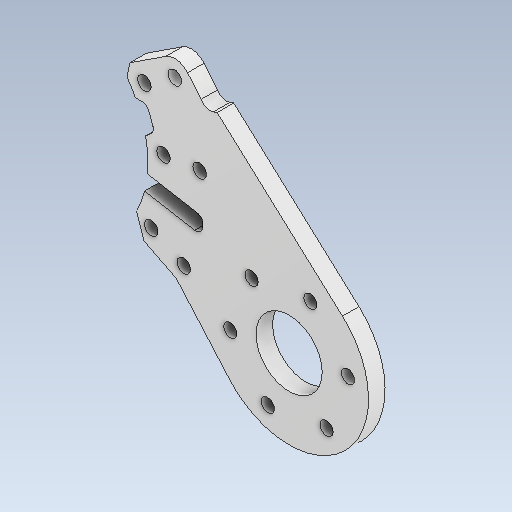
# Autodesk Inventor part: motor_h_5_m
Saved by Autodesk Inventor 2020 (Build 240168000, 168)
## iProperties
Created: 2020-08-09
Part Number: motor_h_5_m
Material: ABS Plastic
Document SubType Name: Modeling
Designer: psrobotics
Density: 1.06 g/cm^3
Appearance: Smooth - White
Author: psrobotics
Autodesk Inventor part; units mm, degrees
ref_plane "YZ Plane" through (0, 0, 0) normal (1, 0, 0) x (0, 1, 0)
ref_plane "XZ Plane" through (0, 0, 0) normal (0, 1, 0) x (-1, 0, 0)
ref_plane "XY Plane" through (0, 0, 0) normal (0, 0, 1) x (1, 0, 0)
sketch "Sketch1" plane through (0, 0, 0) normal (0, 0, 1) x (1, 0, 0)
  circle A0 centre (38.293295, 9.815487) radius 2
  circle A1 centre (49.630187, -4.165746) radius 2
  circle A2 centre (43.190531, -20.974399) radius 2
  circle A3 centre (25.413982, -23.801819) radius 2
  circle A4 centre (14.077089, -9.820586) radius 2
  circle A5 centre (20.516746, 6.988067) radius 2
  circle A6 centre (-68.06383, 51.925322) radius 2.05
  circle A7 centre (-53.750024, 56.410289) radius 2.05
  circle A8 centre (-39.436217, 60.895257) radius 2.05
  line L0 (-78.674955, 0.620135) -> (-78.625805, -1.541882)
  arc A9 (-81.821918, -3.189859) -> (-78.625805, -1.541882) centre (-80.625288, -1.587337) ccw
  line L1 (-81.821918, -3.189859) -> (-83.791584, -1.719076)
  arc A10 (-83.272261, 1.765269) -> (-83.791584, -1.719076) centre (-82.594954, -0.116554) ccw
  line L2 (-83.272261, 1.765269) -> (-81.351745, 2.456502)
  arc A11 (-78.674955, 0.620135) -> (-81.351745, 2.456502) centre (-80.674438, 0.574679) ccw
  line L3 (-1.403552, -3.334837) -> (-3.616041, -5.971578)
  arc A12 (-7.147613, -4.640548) -> (-3.616041, -5.971578) centre (-5.148129, -4.686003) ccw
  line L4 (-7.147613, -4.640548) -> (-7.068079, -1.142036)
  arc A13 (-4.319383, 0.666876) -> (-7.068079, -1.142036) centre (-5.068596, -1.187492) ccw
  line L5 (-4.319383, 0.666876) -> (-2.186427, -0.194894)
  arc A14 (-1.403552, -3.334837) -> (-2.186427, -0.194894) centre (-2.935641, -2.049262) ccw
  arc A15 (-3.40999, 48.096726) -> (-8.055894, 53.961981) centre (-42.851487, 21.62753) ccw
  arc A16 (-4.401032, 43.826911) -> (-3.40999, 48.096726) centre (-5.901032, 46.424987) ccw
  line L6 (-4.401032, 43.826911) -> (-10.914048, 40.066619)
  arc A17 (-14.881949, 40.958979) -> (-10.914048, 40.066619) centre (-12.414048, 42.664695) ccw
  arc A18 (-14.881949, 40.958979) -> (-17.367883, 44.134994) centre (-42.851487, 21.62753) ccw
  arc A19 (-17.417463, 48.04931) -> (-17.367883, 44.134994) centre (-15.11933, 46.120947) ccw
  line L7 (-17.417463, 48.04931) -> (-12.551644, 53.848168)
  arc A20 (-8.055894, 53.961981) -> (-12.551644, 53.848168) centre (-10.25351, 51.919805) ccw
  arc A21 (2.289134, 6.843271) -> (4.050714, 14.115304) centre (-42.851487, 21.62753) ccw
  arc A22 (-1.685672, 4.995462) -> (2.289134, 6.843271) centre (-0.561853, 7.777013) ccw
  line L8 (-1.685672, 4.995462) -> (-8.658636, 7.812722)
  arc A23 (-10.39833, 11.488862) -> (-8.658636, 7.812722) centre (-7.534816, 10.594273) ccw
  arc A24 (-10.39833, 11.488862) -> (-9.42609, 15.403155) centre (-42.851487, 21.62753) ccw
  arc A25 (-6.372092, 17.852118) -> (-9.42609, 15.403155) centre (-6.47679, 14.853945) ccw
  line L9 (-6.372092, 17.852118) -> (1.193168, 17.587933)
  arc A26 (4.050714, 14.115304) -> (1.193168, 17.587933) centre (1.08847, 14.589761) ccw
  line L10 (-77.55058, 9.138616) -> (-84.626781, 6.591747)
  arc A27 (-88.527544, 8.591129) -> (-84.626781, 6.591747) centre (-85.642741, 9.41448) ccw
  arc A28 (-90.338505, 22.73799) -> (-88.527544, 8.591129) centre (-42.851487, 21.62753) ccw
  arc A29 (-87.067158, 25.655485) -> (-90.338505, 22.73799) centre (-87.339325, 22.667856) ccw
  line L11 (-87.067158, 25.655485) -> (-79.577588, 24.973201)
  arc A30 (-76.849895, 21.956541) -> (-79.577588, 24.973201) centre (-79.849755, 21.985572) ccw
  arc A31 (-76.849895, 21.956541) -> (-75.670724, 12.745094) centre (-42.851487, 21.62753) ccw
  arc A32 (-77.55058, 9.138616) -> (-75.670724, 12.745094) centre (-78.566539, 11.96135) ccw
  line L12 (1.367666, 22.584887) -> (-6.197594, 22.849072)
  arc A33 (-9.073322, 25.505106) -> (-6.197594, 22.849072) centre (-6.092896, 25.847245) ccw
  arc A34 (-9.073322, 25.505106) -> (-9.770146, 29.477684) centre (-42.851487, 21.62753) ccw
  arc A35 (-7.778256, 33.023514) -> (-9.770146, 29.477684) centre (-6.851205, 30.170344) ccw
  line L13 (-7.778256, 33.023514) -> (-0.625756, 35.347502)
  arc A36 (3.210472, 33.226926) -> (-0.625756, 35.347502) centre (0.301295, 32.494333) ccw
  arc A37 (4.460489, 25.849725) -> (3.210472, 33.226926) centre (-42.851487, 21.62753) ccw
  arc A38 (1.367666, 22.584887) -> (4.460489, 25.849725) centre (1.472364, 25.58306) ccw
  line L14 (-78.07943, 32.535875) -> (-85.263481, 34.760419)
  arc A39 (-87.175511, 38.704735) -> (-85.263481, 34.760419) centre (-84.376099, 37.626174) ccw
  arc A40 (-83.421221, 46.332726) -> (-87.175511, 38.704735) centre (-42.851487, 21.62753) ccw
  arc A41 (-79.129404, 47.223677) -> (-83.421221, 46.332726) centre (-80.858922, 44.772398) ccw
  line L15 (-79.129404, 47.223677) -> (-72.984388, 42.888016)
  arc A42 (-72.130466, 38.911666) -> (-72.984388, 42.888016) centre (-74.713906, 40.436737) ccw
  arc A43 (-72.130466, 38.911666) -> (-74.407679, 34.284812) centre (-42.851487, 21.62753) ccw
  arc A44 (-78.07943, 32.535875) -> (-74.407679, 34.284812) centre (-77.192048, 35.401631) ccw
  line L16 (-16.381866, 57.062106) -> (-21.247685, 51.263248)
  arc A45 (-25.111143, 50.632361) -> (-21.247685, 51.263248) centre (-23.545819, 53.191611) ccw
  arc A46 (-25.111143, 50.632361) -> (-28.670585, 52.52902) centre (-42.851487, 21.62753) ccw
  arc A47 (-30.238407, 56.281682) -> (-28.670585, 52.52902) centre (-27.419329, 55.255622) ccw
  line L17 (-30.238407, 56.281682) -> (-27.666216, 63.348719)
  arc A48 (-23.633362, 65.06615) -> (-27.666216, 63.348719) centre (-24.847138, 62.322658) ccw
  arc A49 (-17.050461, 61.509319) -> (-23.633362, 65.06615) centre (-42.851487, 21.62753) ccw
  arc A50 (-16.381866, 57.062106) -> (-17.050461, 61.509319) centre (-18.679999, 58.990469) ccw
  line L18 (-27.378641, 16.14178) -> (-17.659555, 17.673703)
  arc A51 (-15.959154, 15.878407) -> (-17.659555, 17.673703) centre (-17.426008, 16.191996) ccw
  arc A52 (-19.770492, 6.677023) -> (-15.959154, 15.878407) centre (-42.851487, 21.62753) ccw
  arc A53 (-22.242323, 6.609923) -> (-19.770492, 6.677023) centre (-21.029455, 7.492505) ccw
  line L19 (-22.242323, 6.609923) -> (-28.031522, 14.565587)
  arc A54 (-27.378641, 16.14178) -> (-28.031522, 14.565587) centre (-27.222943, 15.153976) ccw
  line L20 (-35.789544, 6.807565) -> (-27.833879, 1.018366)
  arc A55 (-27.90098, -1.453465) -> (-27.833879, 1.018366) centre (-28.716462, -0.194501) ccw
  arc A56 (-37.102364, -5.264803) -> (-27.90098, -1.453465) centre (-42.851487, 21.62753) ccw
  arc A57 (-38.897659, -3.564402) -> (-37.102364, -5.264803) centre (-37.415952, -3.797948) ccw
  line L21 (-38.897659, -3.564402) -> (-37.365737, 6.154685)
  arc A58 (-35.789544, 6.807565) -> (-37.365737, 6.154685) centre (-36.377932, 5.998987) ccw
  line L22 (-48.337237, 6.154685) -> (-46.805314, -3.564402)
  arc A59 (-48.60061, -5.264803) -> (-46.805314, -3.564402) centre (-48.287022, -3.797948) ccw
  arc A60 (-57.801994, -1.453465) -> (-48.60061, -5.264803) centre (-42.851487, 21.62753) ccw
  arc A61 (-57.869095, 1.018366) -> (-57.801994, -1.453465) centre (-56.986512, -0.194501) ccw
  line L23 (-57.869095, 1.018366) -> (-49.91343, 6.807565)
  arc A62 (-48.337237, 6.154685) -> (-49.91343, 6.807565) centre (-49.325042, 5.998987) ccw
  line L24 (-57.671452, 14.565587) -> (-63.460651, 6.609923)
  arc A63 (-65.932482, 6.677023) -> (-63.460651, 6.609923) centre (-64.673519, 7.492505) ccw
  arc A64 (-69.74382, 15.878407) -> (-65.932482, 6.677023) centre (-42.851487, 21.62753) ccw
  arc A65 (-68.043419, 17.673703) -> (-69.74382, 15.878407) centre (-68.276966, 16.191996) ccw
  line L25 (-68.043419, 17.673703) -> (-58.324333, 16.14178)
  arc A66 (-57.671452, 14.565587) -> (-58.324333, 16.14178) centre (-58.48003, 15.153976) ccw
  line L26 (-58.324333, 27.11328) -> (-68.043419, 25.581358)
  arc A67 (-69.74382, 27.376654) -> (-68.043419, 25.581358) centre (-68.276966, 27.063065) ccw
  arc A68 (-65.932482, 36.578038) -> (-69.74382, 27.376654) centre (-42.851487, 21.62753) ccw
  arc A69 (-63.460651, 36.645138) -> (-65.932482, 36.578038) centre (-64.673519, 35.762555) ccw
  line L27 (-63.460651, 36.645138) -> (-57.671452, 28.689474)
  arc A70 (-58.324333, 27.11328) -> (-57.671452, 28.689474) centre (-58.48003, 28.101085) ccw
  line L28 (-49.91343, 36.447495) -> (-57.869095, 42.236695)
  arc A71 (-57.801994, 44.708525) -> (-57.869095, 42.236695) centre (-56.986512, 43.449562) ccw
  arc A72 (-48.60061, 48.519864) -> (-57.801994, 44.708525) centre (-42.851487, 21.62753) ccw
  arc A73 (-46.805314, 46.819462) -> (-48.60061, 48.519864) centre (-48.287022, 47.053009) ccw
  line L29 (-46.805314, 46.819462) -> (-48.337237, 37.100376)
  arc A74 (-49.91343, 36.447495) -> (-48.337237, 37.100376) centre (-49.325042, 37.256074) ccw
  line L30 (-37.365737, 37.100376) -> (-38.897659, 46.819462)
  arc A75 (-37.102364, 48.519864) -> (-38.897659, 46.819462) centre (-37.415952, 47.053009) ccw
  arc A76 (-27.90098, 44.708525) -> (-37.102364, 48.519864) centre (-42.851487, 21.62753) ccw
  arc A77 (-27.833879, 42.236695) -> (-27.90098, 44.708525) centre (-28.716462, 43.449562) ccw
  line L31 (-27.833879, 42.236695) -> (-35.789544, 36.447495)
  arc A78 (-37.365737, 37.100376) -> (-35.789544, 36.447495) centre (-36.377932, 37.256074) ccw
  line L32 (-28.031522, 28.689474) -> (-22.242323, 36.645138)
  arc A79 (-19.770492, 36.578038) -> (-22.242323, 36.645138) centre (-21.029455, 35.762555) ccw
  arc A80 (-15.959154, 27.376654) -> (-19.770492, 36.578038) centre (-42.851487, 21.62753) ccw
  arc A81 (-17.659555, 25.581358) -> (-15.959154, 27.376654) centre (-17.426008, 27.063065) ccw
  line L33 (-17.659555, 25.581358) -> (-27.378641, 27.11328)
  arc A82 (-28.031522, 28.689474) -> (-27.378641, 27.11328) centre (-27.222943, 28.101085) ccw
  circle A83 centre (-58.851487, 21.62753) radius 2
  circle A84 centre (-26.851487, 21.62753) radius 2
  circle A85 centre (-32.244885, 11.020929) radius 1.5
  circle A86 centre (-53.458089, 32.234132) radius 1.5
  circle A87 centre (-53.458089, 11.020929) radius 1.5
  circle A88 centre (-32.244885, 32.234132) radius 1.5
  circle A89 centre (-42.851487, 5.62753) radius 2
  circle A90 centre (-42.851487, 37.62753) radius 2
  circle A91 centre (-42.851487, 21.62753) radius 12
  circle A92 centre (7.70065, 40.027004) radius 1.55
  circle A93 centre (-84.475204, 56.808721) radius 1.55
  circle A94 centre (-97.005285, 15.494334) radius 1.55
  circle A95 centre (-90.147142, -5.453293) radius 1.55
  circle A96 centre (-95.005612, 37.445154) radius 1.55
  circle A97 centre (-33.50983, 74.606702) radius 1.55
  circle A98 centre (-1.641007, -12.952168) radius 1.55
  line L34 (-73.415646, -10.729473) -> (-73.624099, -1.560071)
  arc A99 (-66.796705, 1.359267) -> (-73.624099, -1.560071) centre (-69.625132, -1.46916) ccw
  line L35 (-66.796705, 1.359267) -> (-54.272781, -11.164658)
  line L36 (-31.937943, -11.672407) -> (-54.272781, -11.164658)
  line L37 (-31.937943, -11.672407) -> (-18.906268, 1.359267)
  arc A100 (-12.078875, -1.560071) -> (-18.906268, 1.359267) centre (-16.077841, -1.46916) ccw
  line L38 (-12.078875, -1.560071) -> (-12.318903, -12.118417)
  line L39 (-8.896198, -12.196228) -> (-12.318903, -12.118417)
  arc A101 (-7.546122, -12.763059) -> (-8.896198, -12.196228) centre (-8.941653, -14.195711) ccw
  line L40 (-4.169882, -16.05182) -> (-7.546122, -12.763059)
  line L41 (-1.14798, -18.587496) -> (-4.169882, -16.05182)
  line L42 (-1.14798, -18.587496) -> (22.104815, -28.923976)
  arc A102 (22.104815, -28.923976) -> (47.979301, 10.782182) centre (31.853638, -6.993166) ccw
  line L43 (47.979301, 10.782182) -> (10.09134, 45.153855)
  line L44 (8.937474, 44.733882) -> (10.09134, 45.153855)
  arc A103 (5.239682, 46.188463) -> (8.937474, 44.733882) centre (7.911414, 47.55296) ccw
  arc A104 (5.239682, 46.188463) -> (-1.114838, 55.891974) centre (-42.851487, 21.62753) ccw
  arc A105 (-1.795079, 57.715969) -> (-1.114838, 55.891974) centre (1.203865, 57.795554) ccw
  line L45 (-14.440683, 68.326891) -> (-1.795079, 57.715969)
  arc A106 (-16.35509, 68.680064) -> (-14.440683, 68.326891) centre (-14.883068, 71.294094) ccw
  arc A107 (-16.35509, 68.680064) -> (-27.014634, 73.253048) centre (-42.851487, 21.62753) ccw
  arc A108 (-29.089232, 76.642077) -> (-27.014634, 73.253048) centre (-26.134808, 76.121132) ccw
  line L46 (-28.876006, 77.85134) -> (-29.089232, 76.642077)
  line L47 (-36.754468, 79.240526) -> (-28.876006, 77.85134)
  line L48 (-37.439477, 75.355644) -> (-36.754468, 79.240526)
  line L49 (-37.858542, 71.195346) -> (-37.439477, 75.355644)
  arc A109 (-39.248649, 69.487857) -> (-37.858542, 71.195346) centre (-39.848472, 71.395791) ccw
  line L50 (-76.775677, 57.689962) -> (-39.248649, 69.487857)
  arc A110 (-78.666553, 58.07042) -> (-76.775677, 57.689962) centre (-77.3755, 59.597896) ccw
  line L51 (-84.105762, 62.667748) -> (-78.666553, 58.07042)
  line L52 (-89.730392, 56.013112) -> (-84.105762, 62.667748)
  line L53 (-87.956721, 54.513969) -> (-89.730392, 56.013112)
  arc A111 (-87.590763, 51.866531) -> (-87.956721, 54.513969) centre (-89.247774, 52.986494) ccw
  arc A112 (-87.590763, 51.866531) -> (-92.550473, 42.746498) centre (-42.851487, 21.62753) ccw
  arc A113 (-94.971639, 41.614769) -> (-92.550473, 42.746498) centre (-94.391176, 43.528682) ccw
  line L54 (-97.194033, 42.288791) -> (-94.971639, 41.614769)
  line L55 (-99.515886, 34.633139) -> (-97.194033, 42.288791)
  line L56 (-97.293492, 33.959118) -> (-99.515886, 34.633139)
  arc A114 (-95.908867, 31.673145) -> (-97.293492, 33.959118) centre (-97.873956, 32.045205) ccw
  arc A115 (-95.908867, 31.673145) -> (-96.850692, 21.334544) centre (-42.851487, 21.62753) ccw
  arc A116 (-98.625591, 19.336397) -> (-96.850692, 21.334544) centre (-98.850663, 21.323693) ccw
  line L57 (-100.933195, 19.075049) -> (-98.625591, 19.336397)
  line L58 (-100.032909, 11.125868) -> (-100.933195, 19.075049)
  line L59 (-97.725305, 11.387216) -> (-100.032909, 11.125868)
  arc A117 (-95.548493, 9.836621) -> (-97.725305, 11.387216) centre (-97.500234, 9.399921) ccw
  arc A118 (-95.548493, 9.836621) -> (-92.318381, -0.029487) centre (-42.851487, 21.62753) ccw
  arc A119 (-93.156696, -2.567219) -> (-92.318381, -0.029487) centre (-94.150488, -0.831599) ccw
  line L60 (-95.172061, -3.721188) -> (-93.156696, -2.567219)
  line L61 (-88.995524, -14.508281) -> (-95.172061, -3.721188)
  line L62 (-82.535958, -10.809624) -> (-88.995524, -14.508281)
  arc A120 (-81.496711, -10.545761) -> (-82.535958, -10.809624) centre (-81.542166, -12.545245) ccw
  line L63 (-73.415646, -10.729473) -> (-81.496711, -10.545761)
  circle A121 centre (0, 0) radius 2.05
  circle A122 centre (-9.820132, 4.956309) radius 2.05
  circle A123 centre (4.81279, 27.294689) radius 2.05
  circle A124 centre (-6.110273, 25.995965) radius 2.05
  circle A125 centre (-2.695753, 47.924241) radius 2.05
  circle A126 centre (-11.898108, 41.897912) radius 2.05
  circle A127 centre (31.853638, -6.993166) radius 24
  line L64 (0, 0) -> (-9.820132, 4.956309) construction
  line L65 (2.252868, 4.463697) -> (-7.567265, 9.420006)
  line L66 (-12.073, 0.492612) -> (-2.252868, -4.463697)
  arc A128 (-2.252868, -4.463697) -> (2.252868, 4.463697) centre (0, 0) ccw
  arc A129 (-7.567265, 9.420006) -> (-12.073, 0.492612) centre (-9.820132, 4.956309) ccw
  line L67 (-13.628948, 58.787181) -> (-11.330815, 56.858819)
  line L68 (-13.628948, 58.787181) -> (-23.832196, 46.627425)
  spline S0 degree 3 poles (-21.534062, 44.699062) (-21.903382, 45.038051) (-22.279634, 45.368174) (-22.661708, 45.688772) (-23.043782, 46.00937) (-23.434225, 46.322581) (-23.832196, 46.627425) knots 0 0 0 0 0.5 0.5 0.5 1 1 1 1
  line L69 (-21.534062, 44.699062) -> (-11.330815, 56.858819)
  line L70 (3.940984, 14.899895) -> (3.42004, 11.945472)
  line L71 (-11.691298, 17.656288) -> (3.940984, 14.899895)
  spline S1 degree 3 poles (-12.212242, 14.701865) (-12.103331, 15.191187) (-12.00556, 15.682104) (-11.918951, 16.17329) (-11.832342, 16.664475) (-11.756315, 17.159214) (-11.691298, 17.656288) knots 0 0 0 0 0.5 0.5 0.5 1 1 1 1
  line L72 (3.42004, 11.945472) -> (-12.212242, 14.701865)
  line L73 (-2.252868, -4.463697) -> (13.793156, -22.798829)
  line L74 (4.81279, 27.294689) -> (-6.110273, 25.995965) construction
  line L75 (4.222461, 32.259718) -> (-6.700602, 30.960994)
  line L76 (-5.519944, 21.030937) -> (5.403119, 22.329661)
  arc A130 (5.403119, 22.329661) -> (4.222461, 32.259718) centre (4.81279, 27.294689) ccw
  arc A131 (-6.700602, 30.960994) -> (-5.519944, 21.030937) centre (-6.110273, 25.995965) ccw
  line L77 (-2.695753, 47.924241) -> (-11.898108, 41.897912) construction
  line L78 (-5.434993, 52.10713) -> (-14.637349, 46.080801)
  line L79 (-9.158868, 37.715023) -> (0.043488, 43.741352)
  arc A132 (0.043488, 43.741352) -> (-5.434993, 52.10713) centre (-2.695753, 47.924241) ccw
  arc A133 (-14.637349, 46.080801) -> (-9.158868, 37.715023) centre (-11.898108, 41.897912) ccw
  circle A134 centre (-42.851487, 21.62753) radius 32
  line L80 (5.239682, 46.188463) -> (1.15286, 51.116134)
  circle A135 centre (-42.851487, 21.62753) radius 48
  line L81 (4.81279, 27.294689) -> (7.000507, 31.790676)
  line L82 (7.000507, 31.790676) -> (42.354681, 14.587568)
  circle A136 centre (-42.851487, 21.62753) radius 50.87741
  point P0 (0, 0)
  point P1 (-4.910066, 2.478155)
  point P2 (-0.648742, 26.645327)
  point P3 (-7.296931, 44.911077)
  point P4 (-16.080997, 39.158671)
  point P5 (-14.283829, 7.209177)
  dimension "d0" = 48
  dimension "d1" = 10
  dimension "d2" = 10
  dimension "d3" = 10
  dimension "d4" = 64
  constraints: 32 end point, 16 point on circle, 15 tangent, 8 centre point, 4 coincident, 3 midpoint, 3 parallel, 1 perpendicular, 6 other
  measures "d0" diameter of A127
  measures "d1" diameter of A129
  measures "d2" diameter of A131
  measures "d3" diameter of A133
  measures "d4" diameter of A134
extrude "Extrusion1" add sketch "Sketch1" along normal blind 5 contours A14 A121 A135 L65 A128 A136 L66 L3 | L3 L66 A135 A121 A14 | A121 A135 A14 | A14 A135 A121 | L66 L4 A13 L5 A14 A121 A135 | A128 A136 L73 | A135 A121 A14 | A14 A121 A135 | L66 A129 A100 A23 L8 A22 L65 A135 A121 A14 L5 A13 L4 | A136 A128 | A128 A136 A130 L82 A127 L73 | A128 L65 A135 L76 A130 A136 | A127 A102 | L65 A22 A21 A26 L9 A25 L71 A134 A131 L76 A135 | A129 A100 | L82 A136 A132 L80 A103 L44 L43 A127 | L65 A129 A23 A24 L72 L70 L71 A25 L9 A26 A21 A22 | A22 L8 A23 A129 L65 | A136 A130 | A130 L76 A135 A123 L81 A136 | L81 A123 A135 L75 A130 | A130 L75 A135 L79 A132 A136 | L76 A131 A34 A33 L12 A38 A123 A135 | A135 A125 A15 L78 | L78 A132 A136 L79 A135 A125 | A134 L72 A24 A23 A129 | L81 A135 A123 | A123 A135 L81 | A136 A132 | A123 A38 A37 A135 | A15 A125 A16 L6 A17 A18 A133 L78 | A135 A125 A16 A15 | A125 A135 | A134 L71 A25 A24 L72 | A135 A123 A37 L75 | L75 A37 A36 L13 A35 A34 A131 A134 A133 L79 A135 | A123 A37 A38 | A38 L12 A33 A34 A131 L75 A37 A123 | A15 A16 A125 | A135 L79 A133 A18 A17 L6 A16 A125 | A24 A25 L71 L70 L72 | L75 A131 A34 A35 L13 A36 A37 | A92 | A122 | A124 | A126
sketch "Sketch2" plane through (0, 0, 5) normal (0, 0, 1) x (1, 0, 0)
  line L0 (-2.252868, -4.463697) -> (13.793156, -22.798829)
  arc A0 (13.793156, -22.798829) -> (47.979301, 10.782182) centre (31.853638, -6.993166) ccw
  line L1 (47.979301, 10.782182) -> (10.09134, 45.153855)
  line L2 (10.09134, 45.153855) -> (8.937474, 44.733882)
  arc A1 (5.239682, 46.188463) -> (8.937474, 44.733882) centre (7.911414, 47.55296) ccw
  line L3 (5.239682, 46.188463) -> (1.15286, 51.116134)
  arc A2 (1.15286, 51.116134) -> (-5.434993, 52.10713) centre (-2.695753, 47.924241) ccw
  line L4 (-5.434993, 52.10713) -> (-14.637349, 46.080801)
  arc A3 (-14.637349, 46.080801) -> (-16.080997, 39.158671) centre (-11.898108, 41.897912) ccw
  arc A4 (-14.283829, 7.209177) -> (-16.080997, 39.158671) centre (-42.851487, 21.62753) ccw
  arc A5 (-14.283829, 7.209177) -> (-12.073, 0.492612) centre (-9.820132, 4.956309) ccw
  line L5 (-12.073, 0.492612) -> (-2.252868, -4.463697)
  circle A6 centre (20.516746, 6.988067) radius 2
  circle A7 centre (43.190531, -20.974399) radius 2
  circle A8 centre (38.293295, 9.815487) radius 2
  circle A9 centre (25.413982, -23.801819) radius 2
  circle A10 centre (49.630187, -4.165746) radius 2
  circle A11 centre (14.077089, -9.820586) radius 2
  line L6 (-14.637349, 46.080801) -> (-18.820238, 43.34156)
  line L7 (-18.820238, 43.34156) -> (-16.080997, 39.158671)
  line L8 (-12.073, 0.492612) -> (-2.252868, -4.463697)
  line L9 (-12.073, 0.492612) -> (-16.536697, 2.74548)
  arc A12 (-14.283829, 7.209177) -> (-12.073, 0.492612) centre (-9.820132, 4.956309) ccw
  line L10 (-16.536697, 2.74548) -> (-14.283829, 7.209177)
  point P0 (0, 0)
  constraints: 8 end point, 2 perpendicular, 2 tangent, 1 point on line
extrude "Extrusion2" add sketch "Sketch2" against normal blind 5 contours L9 L10 A5 | L7 L6 A3
sketch "Sketch3" plane through (0, 0, 5) normal (0, 0, 1) x (1, 0, 0)
  line L0 (3.940984, 14.899895) -> (3.42004, 11.945472)
  line L1 (-11.691298, 17.656288) -> (3.940984, 14.899895)
  spline S0 degree 3 poles (-12.212242, 14.701865) (-12.103331, 15.191187) (-12.00556, 15.682104) (-11.918951, 16.17329) (-11.832342, 16.664475) (-11.756315, 17.159214) (-11.691298, 17.656288) knots 0 0 0 0 0.5 0.5 0.5 1 1 1 1
  line L2 (3.42004, 11.945472) -> (-12.212242, 14.701865)
  line L3 (3.680512, 13.422683) -> (-11.918951, 16.17329)
  line L4 (3.325122, 10.946782) -> (4.193363, 15.870821)
  line L5 (4.193363, 15.870821) -> (-11.563561, 18.649191)
  line L6 (-11.563561, 18.649191) -> (-12.431802, 13.725153)
  line L7 (-12.431802, 13.725153) -> (3.325122, 10.946782)
  line L8 (3.325122, 10.946782) -> (-11.563561, 18.649191) construction
  line L9 (4.193363, 15.870821) -> (-12.431802, 13.725153) construction
  point P0 (0, 0)
  point P1 (-4.119219, 14.797987)
  dimension "d9" = 5
  dimension "d10" = 16
  constraints: 14 end point, 4 midpoint, 3 parallel, 2 perpendicular, 1 other
  measures "d9" distance of L4.start L4.end
  measures "d10" distance of L5.end L4.end
extrude "Extrusion3" cut sketch "Sketch3" against normal blind 5 contours L0 L3 S0 L1 | L0 L2 S0 L3 | L7 L6 L5 L4
sketch "Sketch4" plane through (0, 0, 5) normal (0, 0, 1) x (1, 0, 0)
  line L0 (3.325122, 10.946782) -> (-11.868079, 13.625753)
  arc A0 (-14.283829, 7.209177) -> (-11.868079, 13.625753) centre (-42.851487, 21.62753) ccw
  line L1 (-14.283829, 7.209177) -> (-16.536697, 2.74548)
  line L2 (-16.536697, 2.74548) -> (-2.252868, -4.463697)
  line L3 (-2.252868, -4.463697) -> (13.793156, -22.798829)
  arc A1 (13.793156, -22.798829) -> (47.979301, 10.782182) centre (31.853638, -6.993166) ccw
  line L4 (47.979301, 10.782182) -> (10.09134, 45.153855)
  line L5 (10.09134, 45.153855) -> (8.937474, 44.733882)
  arc A2 (5.239682, 46.188463) -> (8.937474, 44.733882) centre (7.911414, 47.55296) ccw
  line L6 (5.239682, 46.188463) -> (1.15286, 51.116134)
  arc A3 (1.15286, 51.116134) -> (-5.434993, 52.10713) centre (-2.695753, 47.924241) ccw
  line L7 (-5.434993, 52.10713) -> (-18.820238, 43.34156)
  line L8 (-18.820238, 43.34156) -> (-16.080997, 39.158671)
  arc A4 (-10.999838, 18.549792) -> (-16.080997, 39.158671) centre (-42.851487, 21.62753) ccw
  line L9 (-10.999838, 18.549792) -> (4.193363, 15.870821)
  line L10 (4.193363, 15.870821) -> (3.325122, 10.946782)
  circle A5 centre (20.516746, 6.988067) radius 2
  circle A6 centre (43.190531, -20.974399) radius 2
  circle A7 centre (38.293295, 9.815487) radius 2
  circle A8 centre (25.413982, -23.801819) radius 2
  circle A9 centre (49.630187, -4.165746) radius 2
  circle A10 centre (14.077089, -9.820586) radius 2
  circle A11 centre (31.853638, -6.993166) radius 10
  point P0 (0, 0)
  dimension "d13" = 20
  constraints: 1 centre point, 1 coincident
  measures "d13" diameter of A11
extrude "Extrusion4" cut sketch "Sketch4" against normal blind 5 contours A11
chamfer "Chamfer1" distance 3 angle 45 1 edges at (-18.8202, 43.3416, 2.5)
chamfer "Chamfer2" distance 5 angle 45 1 edges at (-16.5367, 2.7455, 2.5)
sketch "Sketch5" plane through (0, 0, 5) normal (0, 0, 1) x (1, 0, 0)
  arc A0 (-123.056636, 58.258939) -> (-131.834596, 55.184097) centre (-110.157595, 7.368225) ccw
  arc A1 (-134.560031, 57.631234) -> (-131.834596, 55.184097) centre (-132.660386, 57.005654) ccw
  arc A2 (-134.560031, 57.631234) -> (-133.715325, 62.417071) centre (-150.707011, 62.948661) ccw
  arc A3 (-131.205689, 64.288251) -> (-133.715325, 62.417071) centre (-131.716303, 62.354531) ccw
  line L0 (-131.205689, 64.288251) -> (-123.037414, 62.131353)
  arc A4 (-123.056636, 58.258939) -> (-123.037414, 62.131353) centre (-123.548028, 60.197633) ccw
  arc A5 (-157.442017, 47.339699) -> (-150.572417, 45.949194) centre (-150.707011, 62.948661) ccw
  arc A6 (-149.074051, 42.606833) -> (-150.572417, 45.949194) centre (-150.556582, 43.949256) ccw
  arc A7 (-149.074051, 42.606833) -> (-155.546994, 33.751031) centre (-110.157595, 7.368225) ccw
  arc A8 (-159.268211, 34.57847) -> (-155.546994, 33.751031) centre (-157.276114, 34.756091) ccw
  line L1 (-159.268211, 34.57847) -> (-160.226468, 45.325729)
  arc A9 (-157.442017, 47.339699) -> (-160.226468, 45.325729) centre (-158.234371, 45.50335) ccw
  circle A10 centre (-161.555309, 56.082067) radius 2.05
  circle A11 centre (-143.840417, 52.100363) radius 2.05
  circle A12 centre (-139.858714, 69.815255) radius 2.05
  circle A13 centre (-157.573606, 73.796959) radius 2.05
  circle A14 centre (-153.448196, 50.752928) radius 1.55
  circle A15 centre (-147.965827, 75.144394) radius 1.55
  circle A16 centre (-138.511278, 60.207476) radius 1.55
  circle A17 centre (-162.902745, 65.689846) radius 1.55
  line L2 (-72.932848, 48.90084) -> (-57.982009, 44.952951)
  arc A18 (-57.312161, 41.404763) -> (-57.982009, 44.952951) centre (-58.492624, 43.019231) ccw
  arc A19 (-57.312161, 41.404763) -> (-60.282216, 38.844373) centre (-42.851487, 21.62753) ccw
  arc A20 (-63.182513, 38.051978) -> (-60.282216, 38.844373) centre (-62.416591, 40.952558) ccw
  line L3 (-63.182513, 38.051978) -> (-67.8674, 39.28906)
  arc A21 (-70.412507, 40.899226) -> (-67.8674, 39.28906) centre (-66.590864, 44.12336) ccw
  arc A22 (-70.412507, 40.899226) -> (-74.803245, 45.500494) centre (-110.157595, 7.368225) ccw
  arc A23 (-72.932848, 48.90084) -> (-74.803245, 45.500494) centre (-73.443462, 46.96712) ccw
  arc A24 (-61.285218, -10.393835) -> (-59.33292, -3.625063) centre (-110.157595, 7.368225) ccw
  arc A25 (-56.393268, -2.307176) -> (-59.33292, -3.625063) centre (-57.378125, -4.047882) ccw
  arc A26 (-56.393268, -2.307176) -> (-51.935929, -4.328643) centre (-42.851487, 21.62753) ccw
  arc A27 (-51.434594, -7.844156) -> (-51.935929, -4.328643) centre (-52.596616, -6.216364) ccw
  line L4 (-51.434594, -7.844156) -> (-58.243489, -12.704782)
  arc A28 (-61.285218, -10.393835) -> (-58.243489, -12.704782) centre (-59.405511, -11.076991) ccw
  circle A29 centre (-33.553885, 41.566302) radius 2.05
  circle A30 centre (-62.790258, 30.925132) radius 2.05
  circle A31 centre (-52.149089, 1.688759) radius 2.05
  circle A32 centre (-22.912716, 12.329929) radius 2.05
  circle A33 centre (-122.216123, 14.387909) radius 2.1
  circle A34 centre (-150.825947, 7.513846) radius 2.1
  circle A35 centre (-122.266084, 0.435076) radius 2.1
  circle A36 centre (-130.617882, -27.778791) radius 2.1
  circle A37 centre (-110.207556, -6.584608) radius 2.1
  circle A38 centre (-89.94953, -27.924411) radius 2.1
  circle A39 centre (-98.099067, 0.348541) radius 2.1
  circle A40 centre (-69.489243, 7.222605) radius 2.1
  circle A41 centre (-98.049107, 14.301375) radius 2.1
  circle A42 centre (-89.697308, 42.515241) radius 2.1
  circle A43 centre (-130.36566, 42.660861) radius 2.1
  circle A44 centre (-110.107634, 21.321059) radius 2.1
  line L5 (-130.827211, 13.897356) -> (-124.977887, 8.953391)
  arc A45 (-124.988858, 5.889232) -> (-124.977887, 8.953391) centre (-126.26894, 7.425915) ccw
  line L6 (-124.988858, 5.889232) -> (-130.873438, 0.987283)
  arc A46 (-135.746077, 2.760665) -> (-130.873438, 0.987283) centre (-132.79356, 3.292306) ccw
  arc A47 (-135.712425, 12.158914) -> (-135.746077, 2.760665) centre (-110.157595, 7.368225) ccw
  arc A48 (-130.827211, 13.897356) -> (-135.712425, 12.158914) centre (-132.76379, 11.606142) ccw
  line L7 (-126.146796, -7.267622) -> (-118.940535, -4.673941)
  arc A49 (-116.292382, -6.215522) -> (-118.940535, -4.673941) centre (-118.263228, -6.555764) ccw
  line L8 (-116.292382, -6.215522) -> (-114.989459, -13.762692)
  arc A50 (-118.961572, -17.09583) -> (-114.989459, -13.762692) centre (-117.945728, -14.273055) ccw
  arc A51 (-127.083868, -12.367562) -> (-118.961572, -17.09583) centre (-110.157595, 7.368225) ccw
  arc A52 (-126.146796, -7.267622) -> (-127.083868, -12.367562) centre (-125.130836, -10.090356) ccw
  line L9 (-105.47718, -13.796753) -> (-104.120243, -6.259107)
  arc A53 (-101.461118, -4.736529) -> (-104.120243, -6.259107) centre (-102.151884, -6.613453) ccw
  line L10 (-101.461118, -4.736529) -> (-94.273616, -7.38175)
  arc A54 (-93.37309, -12.48827) -> (-94.273616, -7.38175) centre (-95.309764, -10.197136) ccw
  arc A55 (-101.529038, -17.158251) -> (-93.37309, -12.48827) centre (-110.157595, 7.368225) ccw
  arc A56 (-105.47718, -13.796753) -> (-101.529038, -17.158251) centre (-102.524641, -14.328273) ccw
  line L11 (-89.487979, 0.839095) -> (-95.337304, 5.78306)
  arc A57 (-95.326332, 8.847218) -> (-95.337304, 5.78306) centre (-94.046251, 7.310535) ccw
  line L12 (-95.326332, 8.847218) -> (-89.441752, 13.749167)
  arc A58 (-84.569114, 11.975785) -> (-89.441752, 13.749167) centre (-87.521631, 11.444144) ccw
  arc A59 (-84.602766, 2.577537) -> (-84.569114, 11.975785) centre (-110.157595, 7.368225) ccw
  arc A60 (-89.487979, 0.839095) -> (-84.602766, 2.577537) centre (-87.5514, 3.130308) ccw
  line L13 (-94.168394, 22.004072) -> (-101.374656, 19.410391)
  arc A61 (-104.022809, 20.951972) -> (-101.374656, 19.410391) centre (-102.051962, 21.292214) ccw
  line L14 (-104.022809, 20.951972) -> (-105.325732, 28.499142)
  arc A62 (-101.353619, 31.83228) -> (-105.325732, 28.499142) centre (-102.369462, 29.009505) ccw
  arc A63 (-93.231323, 27.104012) -> (-101.353619, 31.83228) centre (-110.157595, 7.368225) ccw
  arc A64 (-94.168394, 22.004072) -> (-93.231323, 27.104012) centre (-95.184354, 24.826806) ccw
  line L15 (-114.83801, 28.533203) -> (-116.194947, 20.995557)
  arc A65 (-118.854072, 19.47298) -> (-116.194947, 20.995557) centre (-118.163307, 21.349903) ccw
  line L16 (-118.854072, 19.47298) -> (-126.041575, 22.1182)
  arc A66 (-126.9421, 27.22472) -> (-126.041575, 22.1182) centre (-125.005427, 24.933586) ccw
  arc A67 (-118.786152, 31.894701) -> (-126.9421, 27.22472) centre (-110.157595, 7.368225) ccw
  arc A68 (-114.83801, 28.533203) -> (-118.786152, 31.894701) centre (-117.790549, 29.064723) ccw
  arc A69 (-78.05356, -25.576136) -> (-65.65721, -4.281482) centre (-110.157595, 7.368225) ccw
  arc A70 (-83.962793, -25.217544) -> (-78.05356, -25.576136) centre (-80.845216, -22.711409) ccw
  line L17 (-83.962793, -25.217544) -> (-87.995212, -20.201301)
  arc A71 (-87.7275, -16.150721) -> (-87.995212, -20.201301) centre (-85.657029, -18.3217) ccw
  arc A72 (-87.7275, -16.150721) -> (-78.630248, -0.523313) centre (-110.157595, 7.368225) ccw
  arc A73 (-75.240121, 1.709603) -> (-78.630248, -0.523313) centre (-75.720031, -1.251763) ccw
  line L18 (-75.240121, 1.709603) -> (-68.886928, 0.680023)
  arc A74 (-65.65721, -4.281482) -> (-68.886928, 0.680023) centre (-69.526808, -3.268464) ccw
  arc A75 (-65.574924, 18.698954) -> (-77.81846, 40.081836) centre (-110.157595, 7.368225) ccw
  arc A76 (-68.84009, 13.760705) -> (-65.574924, 18.698954) centre (-69.451678, 17.713673) ccw
  line L19 (-68.84009, 13.760705) -> (-75.200494, 12.776648)
  arc A77 (-78.574543, 15.033785) -> (-75.200494, 12.776648) centre (-75.659184, 15.741375) ccw
  arc A78 (-78.574543, 15.033785) -> (-87.559649, 30.72594) centre (-110.157595, 7.368225) ccw
  arc A79 (-87.798348, 34.778334) -> (-87.559649, 30.72594) centre (-85.473685, 32.882036) ccw
  line L20 (-87.798348, 34.778334) -> (-83.730109, 39.76557)
  arc A80 (-77.81846, 40.081836) -> (-83.730109, 39.76557) centre (-80.630559, 37.237174) ccw
  arc A81 (-97.678959, 51.643316) -> (-122.318846, 51.731543) centre (-110.157595, 7.368225) ccw
  arc A82 (-95.034892, 46.346474) -> (-97.678959, 51.643316) centre (-98.764057, 47.793308) ccw
  line L21 (-95.034892, 46.346474) -> (-97.362876, 40.346175)
  arc A83 (-101.004638, 38.552731) -> (-97.362876, 40.346175) centre (-100.15975, 41.4313) ccw
  arc A84 (-101.004638, 38.552731) -> (-119.086996, 38.617478) centre (-110.157595, 7.368225) ccw
  arc A85 (-122.715822, 40.436956) -> (-119.086996, 38.617478) centre (-119.911249, 41.502024) ccw
  line L22 (-122.715822, 40.436956) -> (-125.000776, 46.453772)
  arc A86 (-122.318846, 51.731543) -> (-125.000776, 46.453772) centre (-121.261345, 47.873863) ccw
  arc A87 (-142.26163, 40.312587) -> (-154.657981, 19.017932) centre (-110.157595, 7.368225) ccw
  arc A88 (-136.352397, 39.953994) -> (-142.26163, 40.312587) centre (-139.469975, 37.447859) ccw
  line L23 (-136.352397, 39.953994) -> (-132.319978, 34.937752)
  arc A89 (-132.587691, 30.887171) -> (-132.319978, 34.937752) centre (-134.658161, 33.058151) ccw
  arc A90 (-132.587691, 30.887171) -> (-141.684942, 15.259763) centre (-110.157595, 7.368225) ccw
  arc A91 (-145.075069, 13.026847) -> (-141.684942, 15.259763) centre (-144.595159, 15.988213) ccw
  line L24 (-145.075069, 13.026847) -> (-151.428262, 14.056427)
  arc A92 (-154.657981, 19.017932) -> (-151.428262, 14.056427) centre (-150.788382, 18.004914) ccw
  arc A93 (-154.740267, -3.962504) -> (-142.49673, -25.345386) centre (-110.157595, 7.368225) ccw
  arc A94 (-151.4751, 0.975746) -> (-154.740267, -3.962504) centre (-150.863512, -2.977223) ccw
  line L25 (-151.4751, 0.975746) -> (-145.114697, 1.959802)
  arc A95 (-141.740648, -0.297335) -> (-145.114697, 1.959802) centre (-144.656006, -1.004925) ccw
  arc A96 (-141.740648, -0.297335) -> (-132.755541, -15.989489) centre (-110.157595, 7.368225) ccw
  arc A97 (-132.516843, -20.041883) -> (-132.755541, -15.989489) centre (-134.841506, -18.145586) ccw
  line L26 (-132.516843, -20.041883) -> (-136.585081, -25.02912)
  arc A98 (-142.49673, -25.345386) -> (-136.585081, -25.02912) centre (-139.684632, -22.500724) ccw
  arc A99 (-122.636232, -36.906865) -> (-97.996345, -36.995093) centre (-110.157595, 7.368225) ccw
  arc A100 (-125.280298, -31.610023) -> (-122.636232, -36.906865) centre (-121.551133, -33.056857) ccw
  line L27 (-125.280298, -31.610023) -> (-122.952314, -25.609725)
  arc A101 (-119.310552, -23.81628) -> (-122.952314, -25.609725) centre (-120.15544, -26.69485) ccw
  arc A102 (-119.310552, -23.81628) -> (-101.228194, -23.881028) centre (-110.157595, 7.368225) ccw
  arc A103 (-97.599369, -25.700506) -> (-101.228194, -23.881028) centre (-100.403942, -26.765574) ccw
  line L28 (-97.599369, -25.700506) -> (-95.314414, -31.717322)
  arc A104 (-97.996345, -36.995093) -> (-95.314414, -31.717322) centre (-99.053845, -33.137413) ccw
  circle A105 centre (-42.851487, 21.62753) radius 16
  circle A106 centre (-110.157595, 7.368225) radius 8
  circle A107 centre (-150.707011, 62.948661) radius 8
  circle A108 centre (-15.600401, 31.546115) radius 1.5
  circle A109 centre (-97.252978, -47.059623) radius 1.5
  circle A110 centre (-132.912068, -44.130529) radius 1.5
  circle A111 centre (-175.18937, 72.572284) radius 1.5
  circle A112 centre (-125.766491, 71.313495) radius 1.5
  circle A113 centre (-151.188459, 89.250148) radius 1.5
  circle A114 centre (-167.244471, 42.491084) radius 1.5
  circle A115 centre (-148.837607, -33.039403) radius 1.5
  circle A116 centre (-116.601728, -48.563527) radius 1.5
  circle A117 centre (-19.286969, 4.257628) radius 1.5
  circle A118 centre (-35.965177, 50.080628) radius 1.5
  line L29 (-46.010148, 47.99734) -> (-120.395282, 67.639332)
  arc A119 (-121.855514, 69.23281) -> (-120.395282, 67.639332) centre (-119.884667, 69.573052) ccw
  line L30 (-121.855514, 69.23281) -> (-122.997993, 75.85061)
  line L31 (-122.997993, 75.85061) -> (-125.243462, 75.462959)
  arc A120 (-127.316345, 76.43483) -> (-125.243462, 75.462959) centre (-125.583704, 77.433805) ccw
  arc A121 (-127.316345, 76.43483) -> (-145.84392, 89.507094) centre (-150.707011, 62.948661) ccw
  arc A122 (-147.454538, 91.134143) -> (-145.84392, 89.507094) centre (-145.483691, 91.474385) ccw
  line L32 (-147.454538, 91.134143) -> (-147.842189, 93.379612)
  line L33 (-147.842189, 93.379612) -> (-155.725575, 92.018646)
  line L34 (-155.725575, 92.018646) -> (-154.86106, 87.010953)
  arc A123 (-156.331915, 84.734217) -> (-154.86106, 87.010953) centre (-156.831907, 86.670711) ccw
  arc A124 (-156.331915, 84.734217) -> (-169.16322, 75.817941) centre (-150.707011, 62.948661) ccw
  arc A125 (-171.809967, 75.233418) -> (-169.16322, 75.817941) centre (-170.803772, 76.961877) ccw
  line L35 (-171.809967, 75.233418) -> (-176.201782, 77.790044)
  line L36 (-176.201782, 77.790044) -> (-180.226564, 70.876208)
  line L37 (-180.226564, 70.876208) -> (-178.257258, 69.729807)
  arc A126 (-177.294043, 67.652887) -> (-178.257258, 69.729807) centre (-179.263453, 68.001348) ccw
  arc A127 (-177.294043, 67.652887) -> (-171.503787, 45.729656) centre (-150.707011, 62.948661) ccw
  arc A128 (-171.31583, 43.447979) -> (-171.503787, 45.729656) centre (-173.044289, 44.454174) ccw
  line L38 (-171.31583, 43.447979) -> (-172.462231, 41.478672)
  line L39 (-172.462231, 41.478672) -> (-166.442424, 37.974335)
  arc A129 (-165.456522, 36.423497) -> (-166.442424, 37.974335) centre (-167.448619, 36.245876) ccw
  line L40 (-165.456522, 36.423497) -> (-162.450143, 2.705671)
  arc A130 (-162.450143, 2.705671) -> (-156.644264, -17.029308) centre (-110.157595, 7.368225) ccw
  arc A131 (-157.421393, -19.694358) -> (-156.644264, -17.029308) centre (-158.415185, -17.958738) ccw
  line L41 (-157.421393, -19.694358) -> (-161.855253, -22.233123)
  line L42 (-161.855253, -22.233123) -> (-151.996516, -34.848076)
  arc A132 (-151.996516, -34.848076) -> (-148.157913, -38.333932) centre (-110.157595, 7.368225) ccw
  line L43 (-148.157913, -38.333932) -> (-147.537231, -37.587451)
  arc A133 (-144.774025, -37.285473) -> (-147.537231, -37.587451) centre (-145.999386, -38.866135) ccw
  arc A134 (-144.774025, -37.285473) -> (-137.482584, -42.084732) centre (-110.157595, 7.368225) ccw
  arc A135 (-136.667248, -44.742123) -> (-137.482584, -42.084732) centre (-138.44984, -43.83528) ccw
  line L44 (-136.667248, -44.742123) -> (-137.272998, -45.932853)
  arc A136 (-137.272998, -45.932853) -> (-131.552977, -48.475196) centre (-110.157595, 7.368225) ccw
  line L45 (-131.552977, -48.475196) -> (-119.973062, -51.622508)
  arc A137 (-119.973062, -51.622508) -> (-113.753081, -52.325346) centre (-110.157595, 7.368225) ccw
  line L46 (-113.753081, -52.325346) -> (-113.672759, -50.991809)
  arc A138 (-111.624453, -49.11273) -> (-113.672759, -50.991809) centre (-111.676377, -51.112056) ccw
  arc A139 (-111.624453, -49.11273) -> (-102.906817, -48.664589) centre (-110.157595, 7.368225) ccw
  arc A140 (-100.676624, -50.323726) -> (-102.906817, -48.664589) centre (-102.650152, -50.648051) ccw
  line L47 (-100.676624, -50.323726) -> (-100.519194, -51.28169)
  arc A141 (-100.519194, -51.28169) -> (-95.444195, -50.218468) centre (-110.157595, 7.368225) ccw
  line L48 (-95.444195, -50.218468) -> (-80.556247, -44.329432)
  line L49 (-80.556247, -44.329432) -> (-83.095012, -39.895573)
  arc A142 (-82.416207, -37.203799) -> (-83.095012, -39.895573) centre (-81.359392, -38.901781) ccw
  arc A143 (-82.416207, -37.203799) -> (-79.654519, -35.3613) centre (-110.157595, 7.368225) ccw
  line L50 (-79.654519, -35.3613) -> (-28.734972, 0.988339)
  arc A144 (-21.062311, 0.402921) -> (-28.734972, 0.988339) centre (-25.248906, -3.895035) ccw
  line L51 (-21.062311, 0.402921) -> (-19.212728, -1.398739)
  line L52 (-19.212728, -1.398739) -> (-15.026134, 2.899217)
  line L53 (-15.026134, 2.899217) -> (-15.063254, 5.727401)
  line L54 (-15.063254, 5.727401) -> (-16.629101, 7.252675)
  arc A145 (-17.04458, 9.533996) -> (-16.629101, 7.252675) centre (-15.233569, 8.685327) ccw
  arc A146 (-17.04458, 9.533996) -> (-14.676012, 25.916191) centre (-42.851487, 21.62753) ccw
  arc A147 (-13.382826, 28.096535) -> (-14.676012, 25.916191) centre (-12.698786, 26.217149) ccw
  line L55 (-13.382826, 28.096535) -> (-12.352935, 28.471384)
  line L56 (-12.352935, 28.471384) -> (-11.15759, 31.03481)
  line L57 (-11.15759, 31.03481) -> (-12.525671, 34.79358)
  line L58 (-12.525671, 34.79358) -> (-15.089096, 35.988925)
  line L59 (-15.089096, 35.988925) -> (-16.118987, 35.614076)
  arc A148 (-18.511123, 36.453072) -> (-16.118987, 35.614076) centre (-16.803027, 37.493461) ccw
  arc A149 (-18.511123, 36.453072) -> (-30.855823, 47.480075) centre (-42.851487, 21.62753) ccw
  arc A150 (-32.003952, 49.494733) -> (-30.855823, 47.480075) centre (-30.014022, 49.294288) ccw
  line L60 (-32.003952, 49.494733) -> (-31.784872, 51.669668)
  line L61 (-31.784872, 51.669668) -> (-33.574357, 53.860043)
  line L62 (-33.574357, 53.860043) -> (-39.544148, 54.461377)
  line L63 (-39.544148, 54.461377) -> (-39.758787, 52.330528)
  arc A151 (-46.010148, 47.99734) -> (-39.758787, 52.330528) centre (-44.733613, 52.83164) ccw
  line L64 (-12.352935, 28.471384) -> (-7.654472, 30.181485)
  line L65 (-15.089096, 35.988925) -> (-10.390633, 37.699026)
  line L66 (-7.654472, 30.181485) -> (-10.390633, 37.699026)
  point P0 (0, 0)
  dimension "d22" = 5
  dimension "d23" = 5
  constraints: 6 end point, 2 collinear
  measures "d22" distance of L55.end L64.end
  measures "d23" distance of L58.end L65.end
extrude "Extrusion5" cut sketch "Sketch5" against normal blind 5
sketch "Sketch6" plane through (0, 0, 5) normal (0, 0, 1) x (1, 0, 0)
  circle A0 centre (14.077089, -9.820586) radius 2
  circle A1 centre (49.630187, -4.165746) radius 2
  circle A2 centre (25.413982, -23.801819) radius 2
  circle A3 centre (38.293295, 9.815487) radius 2
  circle A4 centre (43.190531, -20.974399) radius 2
  circle A5 centre (20.516746, 6.988067) radius 2
  circle A6 centre (31.853638, -6.993166) radius 10
  line L0 (-14.385252, 36.245104) -> (-10.390633, 37.699026)
  line L1 (-10.390633, 37.699026) -> (-7.654472, 30.181485)
  line L2 (-7.654472, 30.181485) -> (-11.649091, 28.727563)
  arc A7 (-10.999838, 18.549792) -> (-11.649091, 28.727563) centre (-42.851487, 21.62753) ccw
  line L3 (-10.999838, 18.549792) -> (4.193363, 15.870821)
  line L4 (4.193363, 15.870821) -> (3.325122, 10.946782)
  line L5 (3.325122, 10.946782) -> (-11.868079, 13.625753)
  arc A8 (-14.283829, 7.209177) -> (-11.868079, 13.625753) centre (-42.851487, 21.62753) ccw
  line L6 (-12.073, 0.492612) -> (-14.283829, 7.209177)
  line L7 (-12.073, 0.492612) -> (-2.252868, -4.463697)
  line L8 (-2.252868, -4.463697) -> (13.793156, -22.798829)
  arc A9 (13.793156, -22.798829) -> (47.979301, 10.782182) centre (31.853638, -6.993166) ccw
  line L9 (47.979301, 10.782182) -> (10.09134, 45.153855)
  line L10 (10.09134, 45.153855) -> (8.937474, 44.733882)
  arc A10 (5.239682, 46.188463) -> (8.937474, 44.733882) centre (7.911414, 47.55296) ccw
  line L11 (5.239682, 46.188463) -> (1.15286, 51.116134)
  arc A11 (1.15286, 51.116134) -> (-5.434993, 52.10713) centre (-2.695753, 47.924241) ccw
  line L12 (-5.434993, 52.10713) -> (-16.310505, 44.985104)
  line L13 (-17.176694, 40.831827) -> (-16.310505, 44.985104)
  arc A12 (-14.385252, 36.245104) -> (-16.080997, 39.158671) centre (-42.851487, 21.62753) ccw
  line L14 (-7.654472, 30.181485) -> (-11.323397, 27.102891)
  line L15 (-14.385252, 36.245104) -> (-10.390633, 37.699026)
  line L16 (-10.390633, 37.699026) -> (-15.180075, 37.699026)
  line L17 (-17.176694, 40.831827) -> (-16.080997, 39.158671)
  point P0 (0, 0)
  dimension "d26" = 20
  dimension "d27" = 20
  constraints: 4 end point, 2 point on circle
  measures "d26" angle of L0 L16
  measures "d27" angle of L2 L14
extrude "Extrusion6" cut sketch "Sketch6" against normal blind 5 contours A12 L16 L0 | L14 A7 L2
sketch "Sketch7" plane through (0, 0, 5) normal (0, 0, 1) x (1, 0, 0)
  circle A0 centre (-9.820132, 4.956309) radius 2.05
  circle A1 centre (-6.110273, 25.995965) radius 2.05
  circle A2 centre (4.81279, 27.294689) radius 2.05
  circle A3 centre (0, 0) radius 2.05
  circle A4 centre (-11.898108, 41.897912) radius 2.05
  circle A5 centre (-2.695753, 47.924241) radius 2.05
  point P0 (0, 0)
extrude "Extrusion7" cut sketch "Sketch7" against normal blind 5
thicken "Thicken1" operation add thickness 1 both sides no extend neighbours yes toward (-0.6427876, 0.7660444, 0) faces at (-10.100422, 28.129089, 3.333333)
thicken "Thicken2" operation add thickness 1 both sides no extend neighbours yes toward (0, -1, 0) faces at (-11.987114, 37.699026, 3.333333)
thicken "Thicken3" operation add thickness 1 both sides no extend neighbours yes toward (-0.9396926, -0.3420201, 0) faces at (-8.687849, 33.020665, 3.333333)
thicken "Thicken4" operation add thickness 2 both sides no extend neighbours yes toward (0.9848078, -0.1736482, 0) faces at (3.614536, 12.588128, 3.333333)
fillet "Fillet1" radius 2 4 edges at (6.163, 15.5235, 2.5) (5.2947, 10.5995, 2.5) (-8.8336, 30.4974, 2.5) (-11.0908, 36.699, 2.5)
body "Solid1"
